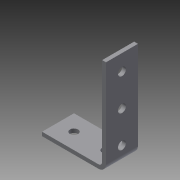
# Autodesk Inventor part: L-Gusset Steel Plate
Saved by Autodesk Inventor 2015 (Build 190159000, 159)
## iProperties
Created: 2015-01-31
Part Number: L-Gusset Steel Plate
Material: Generic
Document SubType Name: Sheet Metal
Designer: chapale16
Density: 1 g/cm^3
Sheet Metal Rule: Default
Appearance: Default
Flat Pattern Width: 2.54 cm
Flat Pattern Length: 12.1702 cm
Flat Pattern Area: 30.9124 cm^2
Sheet Metal Width: 1.000 in
Sheet Metal Length: 4.791 in
Sheet Metal Area: 4.791 in^2
Author: chapale16
Autodesk Inventor part; units mm, degrees
ref_plane "YZ Plane" through (0, 0, 0) normal (1, 0, 0) x (0, 1, 0)
ref_plane "XZ Plane" through (0, 0, 0) normal (0, 1, 0) x (-1, 0, 0)
ref_plane "XY Plane" through (0, 0, 0) normal (0, 0, 1) x (1, 0, 0)
sketch "Sketch1" plane through (0, 0, 0) normal (0, 1, 0) x (-1, 0, 0)
  line L0 (0, 0) -> (0, 25.4)
  line L1 (0, 25.4) -> (50.8, 25.4)
  line L2 (50.8, 25.4) -> (50.8, 0)
  line L3 (50.8, 0) -> (0, 0)
  dimension "d0" = 25.4
  dimension "d1" = 50.8
  measures "d0" distance of L0.start L0.end
  measures "d1" distance of L0.end L1.end
extrude "Plate1" add sketch "Sketch1" along normal blind 3.048
sketch "Sketch2" plane through (-3.048, 0, 0) normal (1, 0, 0) x (0, 1, 0)
  line L0 (0, 25.4) -> (0, 0)
  line L1 (0, 0) -> (76.2, 0)
  line L2 (76.2, 0) -> (76.2, 25.4)
  line L3 (76.2, 25.4) -> (0, 25.4)
  constraints: 6 end point, 1 horizontal, 1 perpendicular, 1 vertical
edge flange "Flange1" height 76.2 angle 90 thickness 3.048 bend radius 3.048 thickness toward (1, 0, 0) relief tear relief width 3.048 relief depth 1.524 edges at (0, 3.048, 12.7) wall of the first edge with corners at (-3.048, 0, 25.4) (-3.048, 0, 0) (-3.048, 76.2, 0) (-3.048, 76.2, 25.4)
bend "Bend1"
corner "Corner1"
hole "Hole1" at (-3.048, 12.7, 12.7) direction (1, 0, 0) diameter 6.35 end through all
pattern_linear "Rectangular Pattern1" count 3 spacing 25.4 along (0, 1, 0) of "Hole1"
hole "Hole2" at (-12.7, 3.048, 12.7) direction (0, -1, 0) diameter 6.35 end through all
pattern_linear "Rectangular Pattern2" count 2 spacing 25.4 along (-1, 0, 0) of "Hole2"
equation "\"d20\" = Thickness"
equation "\"d32\" = Thickness"
equation "\"d3\" = BendReliefWidth"
equation "\"d4\" = BendReliefDepth"
equation "\"d5\" = MinimumRemnant"
equation "\"d6\" = BendRadius"
equation "\"d9\" = BendRadius"
equation "\"d10\" = CornerReliefSize"
equation "\"d11\" = GapSize"
equation "\"d12\" = JacobiRadiusSize"
equation "\"BendRadius\" = Thickness"
equation "\"BendReliefWidth\" = Thickness"
equation "\"BendReliefDepth\" = 0.5 * Thickness"
equation "\"CornerReliefSize\" = 4 * Thickness"
equation "\"MinimumRemnant\" = 2 * Thickness"
equation "\"TransitionRadius\" = BendRadius"
equation "\"JacobiRadiusSize\" = BendRadius"
equation "\"GapSize\" = Thickness"
equation "\"d2\" = BendRadius"
equation "\"Thickness\" = 3.048"
body "Solid1"
